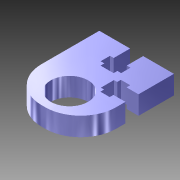
# Autodesk Inventor part: soporte polea eje x
Saved by Autodesk Inventor 2012 SP2 (Build 160219200, 219)
## iProperties
Created: 2014-07-04
Part Number: soporte polea eje x
Material: Default
Document SubType Name: Modeling
Designer: Principal
Density: 1 g/cm^3
Author: Principal
Autodesk Inventor part; units mm, degrees
ref_plane "YZ Plane" through (0, 0, 0) normal (1, 0, 0) x (0, 1, 0)
ref_plane "XZ Plane" through (0, 0, 0) normal (0, 1, 0) x (-1, 0, 0)
ref_plane "XY Plane" through (0, 0, 0) normal (0, 0, 1) x (1, 0, 0)
sketch "Boceto1" plane through (0, 0, 0) normal (0, 0, 1) x (1, 0, 0)
  line L0 (0, 0) -> (20, 0)
  line L1 (20, 0) -> (20, -25)
  line L2 (20, -25) -> (0, -25)
  line L3 (0, -25) -> (0, 0)
  circle A0 centre (10, -18) radius 5
  dimension "d0" = 20
  dimension "d1" = 25
  dimension "d2" = 7
  constraints: 8 end point, 1 centre point
  measures "d0" distance between parallel lines of L1 L3
  measures "d1" distance between parallel lines of L2 L0
  measures "d2" distance from line of A0.centre L2
extrude "Extrusión1" add sketch "Boceto1" along normal blind 5
sketch "Boceto2" plane through (0, 0, 5) normal (0, 0, 1) x (1, 0, 0)
  line L0 (0, 0) -> (20, 0) projected
  line L1 (11.75, -7.9211) -> (8.25, -7.9211)
  line L2 (7.25, -4.3971) -> (7.25, -6.8971)
  line L3 (12.75, -6.8971) -> (12.75, -4.3971)
  line L4 (7.25, -6.8971) -> (8.25, -6.8971)
  line L5 (11.75, -6.8971) -> (12.75, -6.8971)
  line L6 (12.75, -4.3971) -> (11.75, -4.3971)
  line L7 (8.25, -4.3971) -> (7.25, -4.3971)
  line L8 (8.25, -7.9211) -> (8.25, -6.8971)
  line L9 (8.25, -4.3971) -> (8.25, 0)
  line L10 (11.75, 0) -> (11.75, -4.3971)
  line L11 (11.75, -6.8971) -> (11.75, -7.9211)
  constraints: 22 end point, 2 point on line
extrude "Extrusión2" cut sketch "Boceto2" against normal through all
sketch "Boceto3" plane through (0, 0, 5) normal (0, 0, 1) x (1, 0, 0)
  line L0 (20, 0) -> (20, -25) projected
  line L1 (13.4106, -9.5) -> (13.4106, -13)
  line L2 (14.2856, -8.5) -> (16.7856, -8.5)
  line L3 (16.7856, -14) -> (14.2856, -14)
  line L4 (16.7856, -8.5) -> (16.7856, -9.5)
  line L5 (16.7856, -13) -> (16.7856, -14)
  line L6 (14.2856, -14) -> (14.2856, -13)
  line L7 (14.2856, -9.5) -> (14.2856, -8.5)
  line L8 (20, -9.5) -> (16.7856, -9.5)
  line L9 (14.2856, -9.5) -> (13.4106, -9.5)
  line L10 (13.4106, -13) -> (14.2856, -13)
  line L11 (16.7856, -13) -> (20, -13)
  dimension "d12" = 5.5
  constraints: 22 end point, 2 point on line
  measures "d12" distance between parallel lines of L3 L2
extrude "Extrusión3" cut sketch "Boceto3" against normal through all
fillet "Empalme1" radius 9.5 2 edges at (0, -25, 2.5) (20, -25, 2.5)
